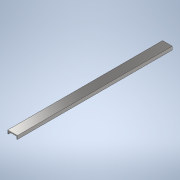
# Autodesk Inventor part: Soporte LED_L=320
Saved by Autodesk Inventor 2020 (Build 240168000, 168)
## iProperties
Created: 2020-08-12
Part Number: Soporte LED_L=320
Material: Stainless Steel, Austenitic
Document SubType Name: Modeling
Designer: Dante
Density: 8 g/cm^3
Appearance: Semi-Polished
Author: Dante
Autodesk Inventor part; units mm, degrees
ref_plane "YZ Plane" through (0, 0, 0) normal (1, 0, 0) x (0, 1, 0)
ref_plane "XZ Plane" through (0, 0, 0) normal (0, 1, 0) x (-1, 0, 0)
ref_plane "XY Plane" through (0, 0, 0) normal (0, 0, 1) x (1, 0, 0)
sketch "Sketch1" plane through (0, 0, 0) normal (0, 0, 1) x (1, 0, 0)
  line L0 (-5.3462, 7.1935) -> (14.6538, 7.1935)
  line L1 (14.6538, 7.1935) -> (14.6538, 0.1935)
  line L2 (14.6538, 0.1935) -> (-5.3462, 0.1935)
  line L3 (-5.3462, 0.1935) -> (-5.3462, 7.1935)
  dimension "d0" = 20
  dimension "d1" = 7
  constraints: 8 end point, 2 parallel, 1 horizontal, 1 perpendicular
  measures "d0" distance of L1.end L2.end
  measures "d1" distance of L0.end L1.end
extrude "Extrusion1" add sketch "Sketch1" along normal blind 320
sketch "Boceto2" plane through (0, 0, 320) normal (0, 0, 1) x (1, 0, 0)
  line L0 (-5.3462, 7.1935) -> (-5.3462, 0.1935) projected
  line L1 (-5.3462, 7.1935) -> (-5.3462, 5.1935)
  line L2 (-5.3462, 5.1935) -> (14.6538, 5.1935)
  line L3 (14.6538, 0.1935) -> (14.6538, 7.1935) projected
  line L4 (-5.3462, 0.1935) -> (-4.3462, 0.1935)
  line L5 (-5.3462, 0.1935) -> (14.6538, 0.1935) projected
  line L6 (-4.3462, 0.1935) -> (-4.3462, 5.1935)
  line L7 (14.6538, 0.1935) -> (13.6538, 0.1935)
  line L8 (13.6538, 0.1935) -> (13.6538, 5.1935)
  line L9 (-4.3462, 0.1935) -> (13.6538, 0.1935)
  point P0 (0, 0)
  dimension "d4" = 2
  dimension "d5" = 1
  dimension "d6" = 1
  constraints: 14 end point, 6 point on line, 4 perpendicular
  measures "d4" distance of L0.start L1.end
  measures "d5" distance of L0.end L4.end
  measures "d6" distance of L3.start L7.end
extrude "Extrusión2" cut sketch "Boceto2" against normal blind 377.5 contours L2 L8 L5 L6
body "Solid1"
